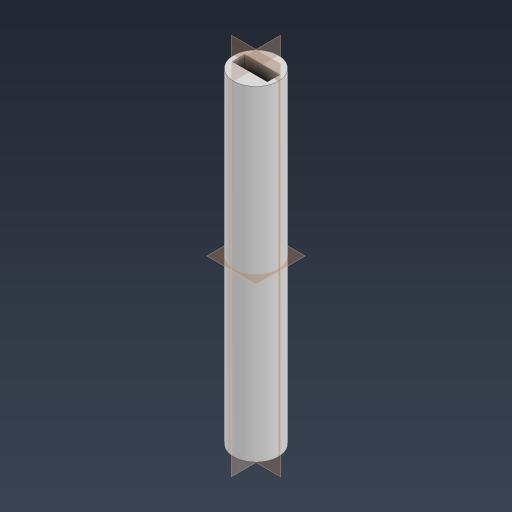
# Autodesk Inventor part: Свеча
Saved by Autodesk Inventor 2023.2 (Build 272271030, 271C)
## iProperties
Created: 2025-11-06
Part Number: Свеча
Material: Типовые
Document SubType Name: Modeling
Designer: Олег Коноваленко
Density: 1 g/cm^3
Appearance: По умолчанию
Author: Олег Коноваленко
Autodesk Inventor part; units mm, degrees
sketch "Эскиз1" plane through (0, 0, 0) normal (0, 0, 1) x (1, 0, 0)
  line L0 (-5.5, 40) -> (-5.5, -40)
  line L1 (-5.5, -40) -> (-4.3, -40)
  line L2 (-4.3, -40) -> (-4.3, -33.7)
  line L3 (-4.3, -33.7) -> (-3.5, -33.7)
  line L4 (-3.5, -33.7) -> (-3.5, 31.5)
  line L5 (-3.5, 31.5) -> (0, 31.5)
  line L6 (0, 31.5) -> (0, 40)
  line L7 (0, 40) -> (-5.5, 40)
  line L8 (0, 56) -> (0, -56) projected
  line L9 (-6.6, 0) -> (1.1, 0) projected
  point P0 (0, 0)
  point P1 (-5.5, 0)
  dimension "d0" = 6.3
  dimension "d1" = 80
  dimension "d2" = 3.5
  dimension "d3" = 8.5
  dimension "d5" = 1.2
  dimension "d6" = 2
  constraints: 16 end point, 6 perpendicular, 2 point on line, 1 midpoint, 1 parallel, 1 vertical
  measures "d0" distance of L1.end L2.end
  measures "d1" distance of L0.start L0.end
  measures "d2" distance between parallel lines of L8 L4
  measures "d3" distance between parallel lines of L5 L7
  measures "d5" distance of L0.end L1.end
  measures "d6" distance between parallel lines of L4 L0
revolve "Вращение1" add sketch "Эскиз1" angle 360 about axis through (0, 0, 0) along (0, -1, 0) contours L7 L6 L5 L4 L9 L0 | L9 L4 L3 L2 L1 L0
sketch "Эскиз2" plane through (0, 40, 0) normal (0, 1, 0) x (1, 0, 0)
  line L0 (-4.3, -1.5) -> (4.3, -1.5)
  line L1 (4.3, -1.5) -> (4.3, 1.5)
  line L2 (4.3, 1.5) -> (-4.3, 1.5)
  line L3 (-4.3, 1.5) -> (-4.3, -1.5)
  line L4 (-4.3, -1.5) -> (4.3, 1.5) construction
  line L5 (4.3, -1.5) -> (-4.3, 1.5) construction
  point P0 (0, 0)
  dimension "d11" = 8.6
  dimension "d12" = 3
  constraints: 12 end point, 2 midpoint, 2 parallel, 1 horizontal, 1 perpendicular
  measures "d11" distance of L1.end L2.end
  measures "d12" distance of L2.end L0.start
extrude "Выдавливание1" cut sketch "Эскиз2" against normal blind 8.5
fillet "Сопряжение1" radius 1 5 edges at (0, 31.5, 3.5) (0, 31.5, -3.5) (-3.4145, 31.5, -0.7688) (-3.4145, 31.5, 0.7688) (3.5, 31.5, 0)
fillet "Сопряжение2" radius 1 6 edges at (0, 31.5, 1.5) (2.8114, 31.2271, 1.5) (-2.8114, 31.2271, 1.5) (-2.8114, 31.2271, -1.5) (2.8114, 31.2271, -1.5) (0, 31.5, -1.5)
